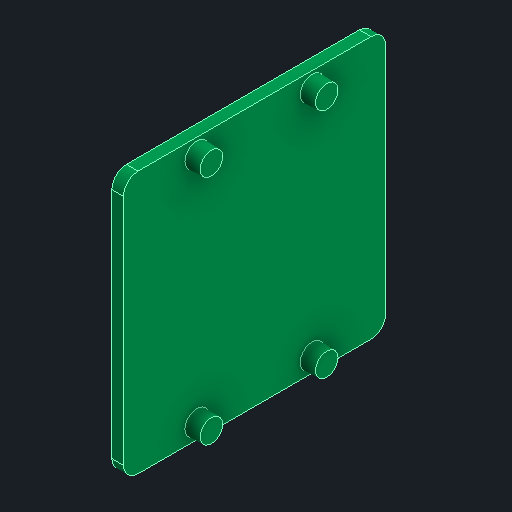
# Autodesk Inventor part: Outer Cover Side
Saved by Autodesk Inventor 2023.4 (Build 274418000, 418)
## iProperties
Created: 2024-07-25
Part Number: Outer Cover Side
Material: Generic
Document SubType Name: Modeling
Designer: xSibe
Density: 1 g/cm^3
Appearance: Plastic Dark Green
Author: xSibe
Autodesk Inventor part; units mm, degrees
ref_plane "YZ Plane" through (0, 0, 0) normal (1, 0, 0) x (0, 1, 0)
ref_plane "XZ Plane" through (0, 0, 0) normal (0, 1, 0) x (-1, 0, 0)
ref_plane "XY Plane" through (0, 0, 0) normal (0, 0, 1) x (1, 0, 0)
ref_plane "Work Plane1" through (-176.5, 0, 24.9) normal (-1, 0, 0) x (0, -1, 0)
sketch "Sketch1" plane through (-176.5, 0, 24.9) normal (-1, 0, 0) x (0, -1, 0)
  arc A0 (20, -22.5) -> (22.5, -20) centre (20, -20) ccw projected
  line L0 (22.5, -20) -> (22.5, 20) projected
  arc A1 (22.5, 20) -> (20, 22.5) centre (20, 20) ccw projected
  line L1 (20, 22.5) -> (-20, 22.5) projected
  arc A2 (-20, 22.5) -> (-22.5, 20) centre (-20, 20) ccw projected
  line L2 (-22.5, 20) -> (-22.5, -20) projected
  arc A3 (-22.5, -20) -> (-20, -22.5) centre (-20, -20) ccw projected
  line L3 (-20, -22.5) -> (20, -22.5) projected
  line L4 (17.25, 10.475) -> (17.25, -7.025) projected
  line L5 (17.25, -7.025) -> (-17.25, -7.025) projected
  line L6 (-17.25, -7.025) -> (-17.25, 10.475) projected
  line L7 (-17.25, 10.475) -> (17.25, 10.475) projected
  point P0 (0, -24.9)
ref_plane "Work Plane2" through (-174.5, -22.5, 2.4) normal (1, 0, 0) x (0, 1, 0)
extrude "Extrusion1" add sketch "Sketch1" against normal up to surface (2 mm away) contours L3 A3 L2 A2 L1 A1 L0 A0 | L4 L5 L6 L7
sketch "Sketch2" plane through (-176.5, 0, 24.9) normal (-1, 0, 0) x (0, 0, 1)
  circle A0 centre (-9.9, -19.9) radius 2.0625 projected
  circle A1 centre (9.9, 19.9) radius 2.0625 projected
  circle A2 centre (-9.9, 19.9) radius 2.0625 projected
  circle A3 centre (9.9, -19.9) radius 2.0625 projected
  arc A4 (-22.5, -20) -> (-20, -22.5) centre (-20, -20) ccw projected
  line L0 (-22.5, 20) -> (-22.5, -20) projected
  arc A5 (-20, 22.5) -> (-22.5, 20) centre (-20, 20) ccw projected
  line L1 (20, 22.5) -> (-20, 22.5) projected
  arc A6 (22.5, 20) -> (20, 22.5) centre (20, 20) ccw projected
  line L2 (22.5, -20) -> (22.5, 20) projected
  arc A7 (20, -22.5) -> (22.5, -20) centre (20, -20) ccw projected
  line L3 (-20, -22.5) -> (20, -22.5) projected
  line L4 (10.475, -17.25) -> (-7.025, -17.25) projected
  line L5 (10.475, 17.25) -> (10.475, -17.25) projected
  line L6 (-7.025, 17.25) -> (10.475, 17.25) projected
  line L7 (-7.025, -17.25) -> (-7.025, 17.25) projected
  point P0 (-24.9, 0)
ref_plane "Work Plane3" through (-172, 17.8375, 32.7375) normal (-1, 0, 0) x (0, 0, 1)
extrude "Extrusion2" add sketch "Sketch2" against normal up to surface (2.5 mm away) from surface at -2 contours A0 | A1 | A2 | A3
chamfer "Chamfer1" distance 0.125 distance2 2.5 1 edges at (-172, 19.9, 32.7375) measured on face at (-172, 19.9, 33.2375)
chamfer "Chamfer2" distance 0.125 distance2 2.5 1 edges at (-172, 19.9, 12.9375) measured on face at (-172, 19.9, 13.4375)
chamfer "Chamfer3" distance 0.125 distance2 2.5 1 edges at (-172, -19.9, 32.7375) measured on face at (-172, -19.9, 33.2375)
chamfer "Chamfer4" distance 0.125 distance2 2.5 1 edges at (-172, -19.9, 12.9375) measured on face at (-172, -19.9, 13.4375)
body "Solid1"
